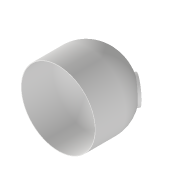
# Autodesk Inventor part: Tank_3
Saved by Autodesk Inventor 2020 (Build 240168000, 168)
## iProperties
Created: 2020-04-08
Part Number: Tank_3
Material: Generisch
Document SubType Name: Modeling
Designer: franz
Density: 1 g/cm^3
Appearance: Vorgabe
Author: franz
Autodesk Inventor part; units mm, degrees
ref_plane "YZ Plane" through (0, 0, 0) normal (1, 0, 0) x (0, 1, 0)
ref_plane "XZ Plane" through (0, 0, 0) normal (0, 1, 0) x (-1, 0, 0)
ref_plane "XY Plane" through (0, 0, 0) normal (0, 0, 1) x (1, 0, 0)
sketch "Skizze1" plane through (0, 0, 0) normal (0, 1, 0) x (-1, 0, 0)
  line L0 (0, -493.487354) -> (0, 702.145893)
  line L1 (0, -500) -> (50, -500)
  line L2 (300, 0) -> (300, -250)
  arc A0 (50, -500) -> (300, -250) centre (50, -250) ccw
  line L3 (300, 0) -> (305, 0)
  line L4 (305, 0) -> (305, -250)
  line L5 (0, -500) -> (0, -505)
  line L6 (0, -505) -> (50, -505)
  arc A1 (50, -505) -> (305, -250) centre (50, -250) ccw
  point P0 (0, 0)
  dimension "d0" = 0
  dimension "d1" = 600
  dimension "d2" = 50
  dimension "d3" = 500
  dimension "d4" = 5
  dimension "d5" = 5
  dimension "d6" = 50
  constraints: 14 end point, 4 point on circle, 4 tangent, 4 vertical, 2 centre point, 2 perpendicular, 1 horizontal, 1 parallel, 1 point on line
  measures "d0" vertical distance of point (0, 0) L2.start
  measures "d1" diameter of L2 L0
  measures "d2" distance of L1.start L1.end
  measures "d3" distance from line of L1 point (0, 0)
  measures "d4" distance between parallel lines of L2 L4
  measures "d5" distance between parallel lines of L1 L6
  measures "d6" distance of L5.end L6.end
revolve "Umdrehung1" add sketch "Skizze1" angle 360 about axis through (0, 0, -493.487354) along (0, 0, 1)
sketch "Skizze2" plane through (0, 0, 0) normal (0, 1, 0) x (-1, 0, 0)
  line L0 (-305, -250) -> (305, -250)
  line L1 (-50, -505) -> (50, -505)
  arc A0 (-305, -250) -> (-50, -505) centre (-50, -250) ccw
  line L2 (-101.948734, -499.652416) -> (-102.850213, -502.129245)
  line L3 (-102.850213, -502.129245) -> (-187.422693, -471.347829)
  line L4 (-187.422693, -471.347829) -> (-185.486683, -466.028607)
  point P0 (0, 0)
  point P1 (-137.214011, -489.622028)
  dimension "d8" = 90
  constraints: 6 end point, 2 perpendicular, 2 point on circle, 1 tangent
  measures "d8" distance of L2.end L3.end
extrude "Extrusion1" add sketch "Skizze2" along normal blind 10
sketch "Skizze3" plane through (137.214011, 0, -489.622028) normal (0.3420157, 0, -0.9396942) x (-0.9396942, 0, -0.3420157)
  line L0 (-53.430873, 0) -> (0, 0)
  circle A0 centre (0, 0) radius 105
  point P0 (-38.519221, 0)
  dimension "d12" = 210
  constraints: 1 centre point
  measures "d12" diameter of A0
extrude "Extrusion2" add sketch "Skizze3" against normal up to surface
sketch "Skizze4" plane through (137.214011, 0, -489.622028) normal (0.3420157, 0, -0.9396942) x (-0.9396942, 0, -0.3420157)
  circle A0 centre (0, 0) radius 100
  point P0 (-38.519221, 0)
  dimension "d15" = 200
  constraints: 1 centre point
  measures "d15" diameter of A0
extrude "Extrusion3" cut sketch "Skizze4" against normal through all
equation "\"d5\" = d4"
equation "\"d6\" = d2"
